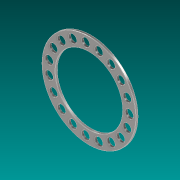
# Autodesk Inventor part: ballRing
Saved by Autodesk Inventor 2020.2 (Build 242310000, 310)
## iProperties
Created: 2020-05-15
Part Number: ballRing
Material: Stainless Steel
Document SubType Name: Modeling
Designer: Svend
Density: 8 g/cm^3
Appearance: Semi-Polished
Author: Svend
Autodesk Inventor part; units mm, degrees
ref_plane "YZ Plane" through (0, 0, 0) normal (1, 0, 0) x (0, 1, 0)
ref_plane "XZ Plane" through (0, 0, 0) normal (0, 1, 0) x (-1, 0, 0)
ref_plane "XY Plane" through (0, 0, 0) normal (0, 0, 1) x (1, 0, 0)
sketch "Sketch1" plane through (0, 0, 0) normal (0, 0, 1) x (1, 0, 0)
  circle A0 centre (0, 0) radius 25
  circle A1 centre (0, 0) radius 35
  circle A2 centre (30, 0) radius 3
  circle A3 centre (28.3745, 9.741) radius 3
  circle A4 centre (23.6742, 18.4264) radius 3
  circle A5 centre (16.4084, 25.115) radius 3
  circle A6 centre (7.3646, 29.082) radius 3
  circle A7 centre (-2.4774, 29.8975) radius 3
  circle A8 centre (-12.0509, 27.4732) radius 3
  circle A9 centre (-20.3184, 22.0717) radius 3
  circle A10 centre (-26.3842, 14.2784) radius 3
  circle A11 centre (-29.5908, 4.9378) radius 3
  circle A12 centre (-29.5908, -4.9378) radius 3
  circle A13 centre (-26.3842, -14.2784) radius 3
  circle A14 centre (-20.3184, -22.0717) radius 3
  circle A15 centre (-12.0509, -27.4732) radius 3
  circle A16 centre (-2.4774, -29.8975) radius 3
  circle A17 centre (7.3646, -29.082) radius 3
  circle A18 centre (16.4084, -25.115) radius 3
  circle A19 centre (23.6742, -18.4264) radius 3
  circle A20 centre (28.3745, -9.741) radius 3
  point P0 (35, 0)
  dimension "d2" = 70
  dimension "d0" = 50
  dimension "d3" = 6
  dimension "d4" = 5
  dimension "d7" = 360
  constraints: 20 centre point, 3 horizontal alignment, 2 coincident, 41 other
  measures "d0" diameter of A0
  measures "d3" diameter of A2
  measures "d4" distance of A2.centre point (35, 0)
extrude "Extrusion1" add sketch "Sketch1" along normal mid plane 1.8
chamfer "Chamfer1" distance 0.2 angle 45 42 edges at (20.6742, -18.4264, -0.9) (13.4084, -25.115, -0.9) (13.4084, -25.115, 0.9) (4.3646, -29.082, 0.9) (-15.0509, -27.4732, -0.9) (-15.0509, -27.4732, 0.9) (-5.4774, -29.8975, -0.9) (-5.4774, -29.8975, 0.9) (20.6742, -18.4264, 0.9) (4.3646, -29.082, -0.9) (25.3745, -9.741, -0.9) (25.3745, -9.741, 0.9) (-25, 0, -0.9) (-25, 0, 0.9) (-35, 0, -0.9) (-35, 0, 0.9) (-29.3842, 14.2784, -0.9) (-29.3842, 14.2784, 0.9) (-23.3184, 22.0717, -0.9) (-23.3184, 22.0717, 0.9) (20.6742, 18.4264, 0.9) (4.3646, 29.082, 0.9) (4.3646, 29.082, -0.9) (20.6742, 18.4264, -0.9) (-29.3842, -14.2784, -0.9) (-29.3842, -14.2784, 0.9) (-23.3184, -22.0717, -0.9) (-23.3184, -22.0717, 0.9) (-32.5908, -4.9378, 0.9) (-32.5908, -4.9378, -0.9) (-32.5908, 4.9378, -0.9) (-32.5908, 4.9378, 0.9) (27, 0, 0.9) (27, 0, -0.9) (-5.4774, 29.8975, -0.9) (-5.4774, 29.8975, 0.9) (13.4084, 25.115, -0.9) (13.4084, 25.115, 0.9) (25.3745, 9.741, -0.9) (25.3745, 9.741, 0.9) (-15.0509, 27.4732, -0.9) (-15.0509, 27.4732, 0.9)
body "Solid1"
